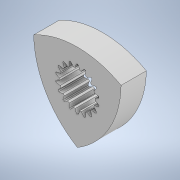
# Autodesk Inventor part: Rotor_Geared
Saved by Autodesk Inventor 2021 (Build 250183000, 183)
## iProperties
Created: 2021-03-24
Part Number: Rotor_Geared
Material: Generic
Document SubType Name: Modeling
Designer: lucia
Density: 1 g/cm^3
Appearance: Default
Author: lucia
Autodesk Inventor part; units mm, degrees
ref_plane "YZ Plane" through (0, 0, 0) normal (1, 0, 0) x (0, 1, 0)
ref_plane "XZ Plane" through (0, 0, 0) normal (0, 1, 0) x (-1, 0, 0)
ref_plane "XY Plane" through (0, 0, 0) normal (0, 0, 1) x (1, 0, 0)
sketch "Sketch1" plane through (0, 0, 0) normal (0, 0, 1) x (1, 0, 0)
  line L0 (0.0008, -101.6013) -> (87.9885, 50.7987)
  line L1 (0.0008, -101.6013) -> (-87.9879, 50.7987)
  line L2 (87.9885, 50.7987) -> (-87.9879, 50.7987)
  line L3 (0.0019, 75.1827) -> (0.0019, 73.5952)
  arc A0 (87.9885, 50.7987) -> (-87.9879, 50.7987) centre (0.0003, -107.6081) ccw
  arc A1 (0.0008, -101.6013) -> (87.9885, 50.7987) centre (-93.1899, 53.8017) ccw
  arc A2 (-87.9879, 50.7987) -> (0.0008, -101.6013) centre (93.1905, 53.8024) ccw
  circle A3 centre (0, 0) radius 39.624
  dimension "d3" = 60
  dimension "d4" = 1.5875
  dimension "d5" = 79.248
  constraints: 8 end point, 7 point on circle, 4 centre point, 2 equal radius, 1 coincident, 1 horizontal, 1 vertical, 6 other
  measures "d3" angle of L1 L0
  measures "d4" distance of L3.start L3.end
  measures "d5" diameter of A3
extrude "Extrusion1" add sketch "Sketch1" against normal blind 50.8
sketch "Sketch2" plane through (0, 0, 0) normal (0, 0, 1) x (1, 0, 0)
  circle A0 centre (0, 0) radius 35.9115
  circle A1 centre (0, 0) radius 39.624
  dimension "d118" = 71.8231
  dimension "d119" = 79.248
  constraints: 2 centre point, 2 coincident
  measures "d118" diameter of A0
  measures "d119" diameter of A1
extrude "Extrusion2" add sketch "Sketch2" against normal blind 50.8
sketch "Sketch3" plane through (0, 0, 0) normal (0, 0, 1) x (1, 0, 0)
  circle A0 centre (0, 0) radius 39.624
  circle A1 centre (0, 0) radius 35.2213
  circle A2 centre (0, 0) radius 35.9115
  circle A3 centre (0, 0) radius 44.0267
  line L0 (0, 0) -> (4.2051, 35.6645)
  line L1 (0, 0) -> (1.3689, 35.8854)
  line L2 (0, 0) -> (-1.4759, 35.8812)
  line L3 (0, 0) -> (-4.3115, 35.6518)
  line L4 (0, 0) -> (-7.1199, 35.1987)
  line L5 (0, 0) -> (-9.8837, 34.5246)
  line L6 (0, 0) -> (-12.5855, 33.634)
  line L7 (0, 0) -> (-15.2083, 32.5322)
  line L8 (0, 0) -> (-17.7357, 31.2263)
  line L9 (0, 0) -> (-20.1517, 29.7245)
  line L10 (4.2051, 35.6645) -> (1.3689, 35.8854)
  line L11 (1.3689, 35.8854) -> (-1.4759, 35.8812)
  line L12 (-1.4759, 35.8812) -> (-4.3115, 35.6518)
  line L13 (-4.3115, 35.6518) -> (-7.1199, 35.1987)
  line L14 (-7.1199, 35.1987) -> (-9.8837, 34.5246)
  line L15 (-9.8837, 34.5246) -> (-12.5855, 33.634)
  line L16 (-12.5855, 33.634) -> (-15.2083, 32.5322)
  line L17 (-15.2083, 32.5322) -> (-17.7357, 31.2263)
  line L18 (-17.7357, 31.2263) -> (-20.1517, 29.7245)
  line L19 (1.3689, 35.8854) -> (4.2116, 35.777)
  line L20 (-1.4759, 35.8812) -> (4.2089, 36.115)
  line L21 (-7.1199, 35.1987) -> (4.0334, 37.4547)
  line L22 (-9.8837, 34.5246) -> (3.7909, 38.4394)
  line L23 (-12.5855, 33.634) -> (3.4008, 39.6159)
  line L24 (-15.2083, 32.5322) -> (2.8314, 40.9655)
  line L25 (-17.7357, 31.2263) -> (2.0536, 42.4661)
  line L26 (-20.1517, 29.7245) -> (1.0404, 44.0917)
  line L27 (-4.3115, 35.6518) -> (4.1612, 36.6764)
  spline S0 degree 4 poles (4.2051, 35.6645) (4.2128, 35.7331) (4.2241, 36.0707) (4.1824, 36.637) (4.0226, 37.5812) (3.7744, 38.5598) (3.2002, 40.2685) (2.4533, 41.8407) (1.6887, 43.1368) (1.0404, 44.0917) knots 0 0 0 0 0 0.159744 0.253879 0.363529 0.486588 0.621664 1 1 1 1 1
  line L28 (0, 0) -> (0, 57.682)
  circle A4 centre (0, 0) radius 39.624 projected
  line L29 (3.4535, 39.4732) -> (0, 0)
  spline S1 degree 4 poles (-4.2051, 35.6645) (-4.2128, 35.7331) (-4.2241, 36.0707) (-4.1824, 36.637) (-4.0226, 37.5812) (-3.7744, 38.5598) (-3.2002, 40.2685) (-2.4533, 41.8407) (-1.6887, 43.1368) (-1.0404, 44.0917) knots 0 0 0 0 0 0.159744 0.253879 0.363529 0.486588 0.621664 1 1 1 1 1
  point P0 (-4.2116, 35.777)
  point P1 (-4.2089, 36.115)
  point P2 (-4.0334, 37.4547)
  point P3 (-3.7909, 38.4394)
  point P4 (-3.4008, 39.6159)
  point P5 (-2.8314, 40.9655)
  point P6 (-2.0536, 42.4661)
  point P7 (-4.1612, 36.6764)
  point P8 (1.0936, 44.0131)
  point P9 (-1.0936, 44.0131)
  point P10 (-4.2051, 35.6645)
  dimension "d87" = 71.8231
  dimension "d84" = 88.0533
  dimension "d85" = 79.248
  dimension "d86" = 70.4427
  dimension "d88" = 2.8448
  dimension "d89" = 2.8448
  dimension "d90" = 5.6896
  dimension "d91" = 8.5344
  dimension "d92" = 11.3792
  dimension "d93" = 14.224
  dimension "d94" = 17.0688
  dimension "d95" = 19.9136
  dimension "d96" = 22.7584
  dimension "d97" = 25.6032
  dimension "d98" = 5
  constraints: 60 end point, 10 symmetric about line, 8 equal length, 4 coincident, 3 centre point, 1 vertical, 44 other
  measures "d84" diameter of A3
  measures "d85" diameter of A0
  measures "d86" diameter of A1
  measures "d88" distance of L0.end L1.end
  measures "d89" distance of L1.end L19.end
  measures "d90" distance of L2.end L20.end
  measures "d91" distance of L3.end L27.end
  measures "d92" distance of L4.end L21.end
  measures "d93" distance of L5.end L22.end
  measures "d94" distance of L6.end L23.end
  measures "d95" distance of L7.end L24.end
  measures "d96" distance of L8.end L25.end
  measures "d97" distance of L9.end L26.end
  measures "d98" angle of L28 L29
extrude "Extrusion3" cut sketch "Sketch3" against normal blind 50.8 contours L29 L22 L28 L23 A0 | A0 L23 S0 | S0 L22 L29 | L23 L28 A0 | A0 L28 L24 S0 L23 | S0 L21 L29 L22 | L29 L21 L28 L22 | S1 L26 L28 L25 A0 | A0 L25 S1 | S1 A3 L28 L26 | L28 L23 S1 L24 A0 | A0 L24 L28 | L28 L22 S1 L23 | S0 L27 L29 L21 | L24 L28 L25 S0 | L28 L21 S1 L22 | L29 L27 L28 L21 | L25 L28 L24 A0 | A0 L24 S1 L25 | L28 A3 L26 | L26 A3 S0 L25 L28 | S0 L20 L29 L27 | L28 L27 S1 L21 | L29 L20 L28 L27 | A2 L29 L19 S0 | S0 L19 L29 L20 | L28 L20 A2 L27 | L29 L19 A2 L28 L20 | A2 L19 L29 | L28 A2 L20
pattern_circular "Circular Pattern1" count 18 over 360 about axis through (0, 0, 0) along (0, 0, -1) of "Extrusion3"
equation "\"prcsn\" = 0.7112"
equation "\"d45\" = 0.5842"
equation "\"d64\" = 0.5842"
equation "\"d83\" = 0.5842"
equation "\"d115\" = 0.7112"
equation "\"d138\" = 0.7112"
body "Solid1"
